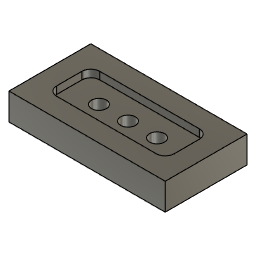
Exam1.1 v3 (Autodesk Fusion 360 design; units mm, degrees)
Autodesk Fusion 360 part; units mm, degrees
sketch "Sketch1" plane through (0, 0, 0) normal (0, 0, 1) x (1, 0, 0)
  line L0 (0, 0) -> (105, 0)
  line L1 (105, 0) -> (105, 55)
  line L2 (105, 55) -> (0, 55)
  line L3 (0, 55) -> (0, 0)
  dimension "d1" = 105
  dimension "d2" = 55
  constraint horizontal L0
  constraint vertical L1
  constraint horizontal L2
  constraint vertical L3
  constraint coincident L0.start L3.end
  measures "d1" distance of L0.start L0.end
  measures "d2" distance of L0 L2
extrude "Extrude1" add sketch "Sketch1" along normal blind 18
sketch "Sketch2" plane through (0, 0, 18) normal (0, 0, 1) x (-1, 0, 0)
  line L0 (0, -55) -> (0, 0)
  line L1 (0, 0) -> (-105, 0)
  line L2 (-105, 0) -> (-105, -55)
  line L3 (-105, -55) -> (0, -55)
  line L4 (0, -55) -> (-105, 0) construction
  line L5 (-105, -55) -> (0, 0) construction
  line L6 (-52.5, -27.5) -> (-52.5, -42) construction
  line L7 (-52.5, -42) -> (-92, -42)
  line L8 (-92, -42) -> (-92, -13)
  line L9 (-92, -13) -> (-13, -13)
  line L10 (-13, -13) -> (-13, -42)
  line L11 (-13, -42) -> (-52.5, -42)
  dimension "d5" = 29
  dimension "d6" = 79
  dimension "d7" = 14.5
  dimension "d8" = 39.5
  constraint coincident L0.start L3.end
  constraint coincident L1.end L2.start
  constraint coincident L2.end L3.start
  constraint coincident L0.end L1.start
  constraint midpoint L5 L6.start
  constraint parallel L0 L6
  constraint perpendicular L0 L7
  constraint perpendicular L7 L8
  constraint perpendicular L8 L9
  constraint perpendicular L9 L10
  constraint perpendicular L6 L11
  measures "d5" distance of L7 L9
  measures "d6" distance of L8 L10
  measures "d7" distance of L6.start L6.end
  measures "d8" distance of L6.start L8
extrude "Extrude2" cut sketch "Sketch2" against normal blind 5 contours L7 L8 L9 L10 L11
fillet "Fillet1" radius 6 4 edges at (13, 42, 15.5) (92, 42, 15.5) (92, 13, 15.5) (13, 13, 15.5)
sketch "Sketch3" plane through (0, 0, 13) normal (0, 0, 1) x (-1, 0, 0)
  arc A0 (-13, -19) -> (-19, -13) centre (-19, -19) ccw
  line L0 (-19, -13) -> (-86, -13)
  arc A1 (-86, -13) -> (-92, -19) centre (-86, -19) ccw
  line L1 (-92, -19) -> (-92, -36)
  arc A2 (-92, -36) -> (-86, -42) centre (-86, -36) ccw
  line L2 (-86, -42) -> (-19, -42)
  arc A3 (-19, -42) -> (-13, -36) centre (-19, -36) ccw
  line L3 (-13, -36) -> (-13, -19)
  line L4 (0, -55) -> (-105, 0) construction
  line L5 (-105, 0) -> (-105, -55) construction
  line L6 (-105, -55) -> (0, 0) construction
  line L7 (-52.5, -27.5) -> (-33, -27.5) construction
  line L8 (-52.5, -27.5) -> (-72, -27.5) construction
  dimension "d13" = 19.5
  dimension "d14" = 19.5
  constraint vertical L5
  constraint coincident L6.end origin
  constraint midpoint L4 L7.start
  constraint parallel L2 L7
  constraint parallel L7 L8
  measures "d13" distance of L7.start L7.end
  measures "d14" distance of L7.start L8.end
hole "Hole1" at (52.5, 27.5, 13) at (72, 27.5, 13) at (33, 27.5, 13) direction (0, 0, -1) diameter 10 depth 10 tip angle 180
equation "d7 = ( 29 / 2 ) * 1 mm"
equation "d8 = ( 79 / 2 ) * 1 mm"
